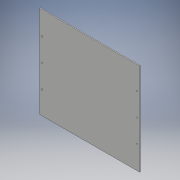
# Autodesk Inventor part: inner_panel
Saved by Autodesk Inventor 2018 (Build 220112000, 112)
## iProperties
Created: 2021-05-01
Part Number: inner_panel
Material: Generic
Document SubType Name: Modeling
Designer: gisen
Density: 1 g/cm^3
Appearance: Default
Author: gisen
Autodesk Inventor part; units mm, degrees
ref_plane "YZ Plane" through (0, 0, 0) normal (1, 0, 0) x (0, 1, 0)
ref_plane "XZ Plane" through (0, 0, 0) normal (0, 1, 0) x (-1, 0, 0)
ref_plane "XY Plane" through (0, 0, 0) normal (0, 0, 1) x (1, 0, 0)
sketch "Sketch1" plane through (0, 0, 0) normal (0, 1, 0) x (-1, 0, 0)
  line L0 (185, 170) -> (-185, 170)
  line L1 (-185, 170) -> (-185, -170)
  line L2 (-185, -170) -> (185, -170)
  line L3 (185, -170) -> (185, 170)
  line L4 (185, 170) -> (-185, -170) construction
  line L5 (-185, 170) -> (185, -170) construction
  point P0 (0, 0)
  dimension "d0" = 340
  dimension "d1" = 370
  constraints: 12 end point, 2 midpoint, 2 parallel, 1 horizontal, 1 perpendicular
  measures "d0" distance of L2.end L0.start
  measures "d1" distance of L1.end L2.end
extrude "Extrusion1" add sketch "Sketch1" along normal blind 3
sketch "Sketch3" plane through (0, 0, 0) normal (0, -1, 0) x (1, 0, 0)
  line L0 (-185, -170) -> (-185, 170) projected
  line L1 (185, -170) -> (-185, -170) projected
  line L2 (-185, 170) -> (185, 170) projected
  point P0 (0, 0)
  point P1 (-175, 0)
  point P2 (-175, -85)
  point P3 (-175, 85)
  point P4 (175, 85)
  point P5 (175, 0)
  point P6 (175, -85)
  dimension "d22" = 10
  dimension "d23" = 170
  dimension "d24" = 10
  dimension "d25" = 85
  dimension "d26" = 10
  dimension "d27" = 85
  dimension "d30" = 360
  constraints: 7 other
  measures "d22" distance from line of L0 point (-175, 0)
  measures "d23" distance from line of L1 point (-175, 0)
  measures "d24" distance from line of point (-175, -85) L0
  measures "d25" distance from line of L1 point (-175, -85)
  measures "d26" distance from line of L0 point (-175, 85)
  measures "d27" distance from line of L2 point (-175, 85)
hole "Hole2" at (-175, 0, 0) at (-175, 0, -85) at (-175, 0, 85) at (175, 0, 85) at (175, 0, 0) at (175, 0, -85) direction (0, 1, 0) diameter 4.5 end through all
equation "\"d24\" = d22"
equation "\"d25\" = 0.5 * d23"
equation "\"d26\" = d22"
equation "\"d27\" = d25"
body "Solid1"
